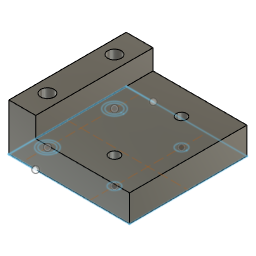
droy-front v4 (Autodesk Fusion 360 design; units mm, degrees)
Autodesk Fusion 360 part; units mm, degrees
sketch "Sketch2" plane through (0, 0, 0) normal (0, 0, 1) x (1, 0, 0)
  line L0 (-0.1454, 35.3341) -> (35.8546, 35.3341)
  line L1 (35.8546, 35.3341) -> (35.8546, 0.3341)
  line L2 (35.8546, 0.3341) -> (-0.1454, 0.3341)
  line L3 (-0.1454, 0.3341) -> (-0.1454, 35.3341)
  line L4 (-0.1454, 17.8341) -> (35.8546, 17.8341) construction
  line L5 (23.8546, 0.3341) -> (23.8546, 35.3341) construction
  circle A0 centre (23.8546, 27.8341) radius 1.55
  circle A1 centre (23.8546, 7.8341) radius 1.55
  line L6 (3.8546, 35.3341) -> (3.8546, 0.3341) construction
  circle A2 centre (3.8546, 27.8341) radius 2
  circle A3 centre (3.8546, 7.8341) radius 2
  circle A4 centre (3.8546, 27.8341) radius 2.7
  circle A5 centre (3.8546, 7.8341) radius 2.7
  line L7 (-0.1454, 0.3341) -> (7.8546, 0.3341)
  line L8 (7.8546, 35.4069) -> (-0.1454, 35.4069)
  line L9 (-0.1454, 35.4069) -> (-0.1454, 0.3341)
  dimension "d22" = 36
  dimension "d23" = 35
  dimension "d24" = 3.1
  dimension "d25" = 3.1
  dimension "d26" = 10
  dimension "d27" = 10
  dimension "d28" = 12
  dimension "d29" = 4
  dimension "d30" = 4
  dimension "d31" = 4
  dimension "d32" = 10
  dimension "d33" = 10
  dimension "d34" = 5.4
  dimension "d35" = 5.4
  dimension "d40" = 8
  constraint horizontal L0
  constraint vertical L1
  constraint horizontal L2
  constraint vertical L3
  constraint midpoint L3 L4.start
  constraint midpoint L1 L4.end
  constraint coincident L2 L5.start
  constraint perpendicular L2 L5
  constraint coincident L0 L5.end
  constraint coincident L5 A0.centre
  constraint coincident L5 A1.centre
  constraint coincident L0 L6.start
  constraint perpendicular L0 L6
  constraint coincident L2 L6.end
  constraint coincident L6 A2.centre
  constraint coincident L6 A3.centre
  constraint concentric A2 A4
  constraint concentric A3 A5
  constraint horizontal L7
  constraint horizontal L8
  constraint vertical L9
  measures "d22" distance of L0.start L0.end
  measures "d23" distance of L0.start L2.end
  measures "d24" diameter of A0
  measures "d25" diameter of A1
  measures "d26" distance of L4 A0.centre
  measures "d27" distance of L4 A1.centre
  measures "d28" distance of L1 L5
  measures "d29" distance of L3 L6
  measures "d30" diameter of A2
  measures "d31" diameter of A3
  measures "d32" distance of L4 A2.centre
  measures "d33" distance of L4 A3.centre
  measures "d34" diameter of A4
  measures "d35" diameter of A5
  measures "d40" distance of L2.end L7.end
extrude "Extrude5" add sketch "Sketch2" along normal blind 8 contours L0 L1 L2 L3 L7 L9 | A4 | A5
extrude "Extrude6" cut sketch "Sketch2" along normal blind 6 contours A4 | A5
sketch "Sketch3" plane through (0, 0, 8) normal (0, 0, 1) x (-1, 0, 0)
  circle A0 centre (-23.8546, -7.8341) radius 1.55
  circle A1 centre (-3.8546, -7.8341) radius 2
  circle A2 centre (-23.8546, -27.8341) radius 1.55
  circle A3 centre (-3.8546, -27.8341) radius 2
  line L0 (0.1454, -0.3341) -> (-35.8546, -0.3341)
  line L1 (-35.8546, -0.3341) -> (-35.8546, -35.3341)
  line L2 (-35.8546, -35.3341) -> (0.1454, -35.3341)
  line L3 (0.1454, -35.3341) -> (0.1454, -0.3341)
  line L4 (0.1454, -0.3341) -> (-7.8546, -0.3341)
  line L5 (-7.8546, -0.3341) -> (-7.8546, -35.3341)
  line L6 (-7.8546, -35.3341) -> (0.1454, -35.3341)
  line L7 (0.1454, -35.3341) -> (0.1454, -0.3341)
  dimension "d45" = 8
  dimension "d46" = 35
  constraint horizontal L4
  constraint vertical L5
  constraint horizontal L6
  constraint vertical L7
  constraint coincident L0.start L3.end
  measures "d45" distance of L0.start L4.end
  measures "d46" distance of L0.start L2.end
extrude "Extrude9" add sketch "Sketch3" along normal blind 6 contours L0 L2 L3 L4 L5 L6 L7
